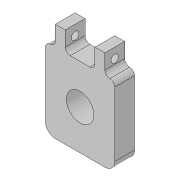
# Autodesk Inventor part: Needle Bearing Mount v2
Saved by Autodesk Inventor 2018.3 (Build 223284000, 284)
## iProperties
Created: 2019-03-08
Part Number: Needle Bearing Mount v2
Material: Generic
Document SubType Name: Modeling
Designer: aye06091
Mass: 27.2141 g
Surface Area: 80.3898 cm^2
Volume: 27.2141 cm^3
Density: 1 g/cm^3
Appearance: Default
Author: aye06091
Autodesk Inventor part; units mm, degrees
ref_plane "YZ Plane" through (0, 0, 0) normal (1, 0, 0) x (0, 1, 0)
ref_plane "XZ Plane" through (0, 0, 0) normal (0, 1, 0) x (-1, 0, 0)
ref_plane "XY Plane" through (0, 0, 0) normal (0, 0, 1) x (1, 0, 0)
sketch "Sketch1" plane through (0, 0, 0) normal (0, 0, 1) x (1, 0, 0)
  line L0 (0, 0) -> (44.45, 0)
  line L1 (44.45, 0) -> (44.45, -50.8)
  line L2 (44.45, -50.8) -> (0, -50.8)
  line L3 (0, -50.8) -> (0, 0)
  line L4 (6.35, 0) -> (12.7, 0)
  line L5 (12.7, 0) -> (12.7, 12.7)
  line L6 (12.7, 12.7) -> (6.35, 12.7)
  line L7 (6.35, 12.7) -> (6.35, 0)
  line L8 (31.75, 0) -> (38.1, 0)
  line L9 (38.1, 0) -> (38.1, 12.7)
  line L10 (38.1, 12.7) -> (31.75, 12.7)
  line L11 (31.75, 12.7) -> (31.75, 0)
  circle A0 centre (22.225, -25.4) radius 9.5885
  dimension "d0" = 44.45
  dimension "d1" = 50.8
  dimension "d3" = 6.35
  dimension "d4" = 6.35
  dimension "d5" = 6.35
  dimension "d6" = 19.05
  dimension "d9" = 19.177
  dimension "d20" = 12.7
  dimension "d21" = 22.225
  dimension "d22" = 25.4
  dimension "d25" = 6.35
  constraints: 24 end point, 6 parallel, 3 horizontal, 3 perpendicular, 3 point on line, 1 centre point
  measures "d0" distance of L0.start L0.end
  measures "d1" distance of L2.end L0.start
  measures "d3" distance between parallel lines of L1 L9
  measures "d4" distance between parallel lines of L9 L11
  measures "d5" distance of L5.end L6.end
  measures "d6" distance between parallel lines of L11 L5
  measures "d9" diameter of A0
  measures "d20" distance of L6.end L4.start
  measures "d21" distance from line of L3 A0.centre
  measures "d22" distance from line of L2 A0.centre
  measures "d25" distance between parallel lines of L3 L7
extrude "Extrusion1" add sketch "Sketch1" against normal blind 12.7 contours L0 L1 L2 L3 | L7 L6 L5 L0 | L11 L10 L9 L0 | A0
sketch "Sketch2" plane through (0, 0, 0) normal (0, 0, 1) x (1, 0, 0)
  circle A0 centre (22.225, -25.4) radius 8.8265
  line L0 (0, -50.8) -> (0, 0) projected
  dimension "d10" = 17.653
  dimension "d23" = 22.225
  constraints: 1 centre point
  measures "d10" diameter of A0
  measures "d23" distance from line of L0 A0.centre
extrude "Extrusion2" cut sketch "Sketch2" against normal blind 12.7
sketch "Sketch3" plane through (38.1, 0, 0) normal (1, 0, 0) x (0, 0, -1)
  line L0 (12.7, 12.7) -> (12.7, 0) projected
  line L1 (0, 12.7) -> (12.7, 12.7) projected
  circle A0 centre (6.35, 6.35) radius 2.4447
  dimension "d13" = 4.8895
  dimension "d14" = 6.35
  dimension "d15" = 6.35
  constraints: 1 centre point
  measures "d13" diameter of A0
  measures "d14" distance from line of L0 A0.centre
  measures "d15" distance from line of L1 A0.centre
extrude "Extrusion3" cut sketch "Sketch3" against normal through all
fillet "Fillet2" radius 6.35 2 edges at (44.45, -50.8, -6.35) (0, -50.8, -6.35)
fillet "Fillet3" radius 3.175 6 edges at (38.1, 0, -6.35) (12.7, 0, -6.35) (31.75, 0, -6.35) (6.35, 0, -6.35) (44.45, 0, -6.35) (0, 0, -6.35)
body "Solid1"
